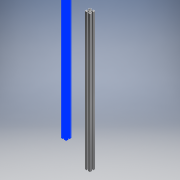
# Autodesk Inventor part: Propile_800
Saved by Autodesk Inventor 2019 (Build 230136000, 136)
## iProperties
Created: 2019-04-15
Part Number: Propile_800
Material: 알루미늄 6061
Document SubType Name: Modeling
Designer: hinmo
Density: 2.7 g/cm^3
Appearance: 알루미늄 - 평지
Mass: 694.099 g
Surface Area: 2965.78 cm^2
Volume: 257.074 cm^3
Author: hinmo
Autodesk Inventor part; units mm, degrees
ref_plane "YZ Plane" through (0, 0, 0) normal (1, 0, 0) x (0, 1, 0)
ref_plane "XZ Plane" through (0, 0, 0) normal (0, 1, 0) x (-1, 0, 0)
ref_plane "XY Plane" through (0, 0, 0) normal (0, 0, 1) x (1, 0, 0)
sketch "스케치1" plane through (0, 0, 0) normal (0, 1, 0) x (-1, 0, 0)
  line L0 (15, 15) -> (-15, -15) construction
  line L1 (-15, 15) -> (15, -15) construction
  line L2 (10, 10) -> (-10, -10) construction
  line L3 (-10, 10) -> (10, -10) construction
  circle A0 centre (-10, -10) radius 3
  arc A1 (-15, -13.5) -> (-13.5, -15) centre (-13.5, -13.5) ccw
  arc A2 (-13.5, 15) -> (-15, 13.5) centre (-13.5, 13.5) ccw
  arc A3 (15, 13.5) -> (13.5, 15) centre (13.5, 13.5) ccw
  arc A4 (13.5, -15) -> (15, -13.5) centre (13.5, -13.5) ccw
  line L4 (-7, -7) -> (-13, -13) construction
  line L5 (-13, -7) -> (-7, -13) construction
  line L6 (-7.5303, -6.4697) -> (-13.5303, -12.4697)
  line L7 (-13.5303, -12.4697) -> (-12.4697, -13.5303)
  line L8 (-12.4697, -13.5303) -> (-6.4697, -7.5303)
  line L9 (-6.4697, -7.5303) -> (-7.5303, -6.4697)
  line L10 (-7.5303, -6.4697) -> (-12.4697, -13.5303) construction
  line L11 (-13.5303, -12.4697) -> (-6.4697, -7.5303) construction
  line L12 (-13.5303, -7.5303) -> (-7.5303, -13.5303)
  line L13 (-7.5303, -13.5303) -> (-6.4697, -12.4697)
  line L14 (-6.4697, -12.4697) -> (-12.4697, -6.4697)
  line L15 (-12.4697, -6.4697) -> (-13.5303, -7.5303)
  line L16 (-13.5303, -7.5303) -> (-6.4697, -12.4697) construction
  line L17 (-7.5303, -13.5303) -> (-12.4697, -6.4697) construction
  circle A5 centre (-10, 10) radius 3
  line L18 (-7, 13) -> (-13, 7) construction
  line L19 (-13, 13) -> (-7, 7) construction
  line L20 (-7.5303, 13.5303) -> (-13.5303, 7.5303)
  line L21 (-13.5303, 7.5303) -> (-12.4697, 6.4697)
  line L22 (-12.4697, 6.4697) -> (-6.4697, 12.4697)
  line L23 (-6.4697, 12.4697) -> (-7.5303, 13.5303)
  line L24 (-7.5303, 13.5303) -> (-12.4697, 6.4697) construction
  line L25 (-13.5303, 7.5303) -> (-6.4697, 12.4697) construction
  line L26 (-13.5303, 12.4697) -> (-7.5303, 6.4697)
  line L27 (-7.5303, 6.4697) -> (-6.4697, 7.5303)
  line L28 (-6.4697, 7.5303) -> (-12.4697, 13.5303)
  line L29 (-12.4697, 13.5303) -> (-13.5303, 12.4697)
  circle A6 centre (10, 10) radius 3
  line L30 (13, 13) -> (7, 7) construction
  line L31 (7, 13) -> (13, 7) construction
  line L32 (12.4697, 13.5303) -> (6.4697, 7.5303)
  line L33 (6.4697, 7.5303) -> (7.5303, 6.4697)
  line L34 (7.5303, 6.4697) -> (13.5303, 12.4697)
  line L35 (13.5303, 12.4697) -> (12.4697, 13.5303)
  line L36 (12.4697, 13.5303) -> (7.5303, 6.4697) construction
  line L37 (6.4697, 7.5303) -> (13.5303, 12.4697) construction
  line L38 (6.4697, 12.4697) -> (12.4697, 6.4697)
  line L39 (12.4697, 6.4697) -> (13.5303, 7.5303)
  line L40 (13.5303, 7.5303) -> (7.5303, 13.5303)
  line L41 (7.5303, 13.5303) -> (6.4697, 12.4697)
  line L42 (6.4697, 12.4697) -> (13.5303, 7.5303) construction
  line L43 (12.4697, 6.4697) -> (7.5303, 13.5303) construction
  circle A7 centre (10, -10) radius 3
  line L44 (13, -7) -> (7, -13) construction
  line L45 (7, -7) -> (13, -13) construction
  line L46 (12.4697, -6.4697) -> (6.4697, -12.4697)
  line L47 (6.4697, -12.4697) -> (7.5303, -13.5303)
  line L48 (7.5303, -13.5303) -> (13.5303, -7.5303)
  line L49 (13.5303, -7.5303) -> (12.4697, -6.4697)
  line L50 (12.4697, -6.4697) -> (7.5303, -13.5303) construction
  line L51 (6.4697, -12.4697) -> (13.5303, -7.5303) construction
  line L52 (6.4697, -7.5303) -> (12.4697, -13.5303)
  line L53 (12.4697, -13.5303) -> (13.5303, -12.4697)
  line L54 (13.5303, -12.4697) -> (7.5303, -6.4697)
  line L55 (7.5303, -6.4697) -> (6.4697, -7.5303)
  line L56 (6.4697, -7.5303) -> (13.5303, -12.4697) construction
  line L57 (12.4697, -13.5303) -> (7.5303, -6.4697) construction
  line L58 (-3.15, -15) -> (-3.15, -12.5)
  line L59 (-3.15, -12.5) -> (-5.1, -12.5)
  line L60 (0, -4.5) -> (-3.435, -4.5)
  arc A8 (-3.435, -4.5) -> (-6.0787, -8.8068) centre (0.5972, -9.94) ccw
  line L61 (-5.1, -12.5) -> (-6.0787, -8.8068)
  line L62 (3.15, -15) -> (3.15, -12.5)
  line L63 (3.15, -12.5) -> (5.1, -12.5)
  line L64 (0, -4.5) -> (3.435, -4.5)
  arc A9 (6.0787, -8.8068) -> (3.435, -4.5) centre (-0.5972, -9.94) ccw
  line L65 (5.1, -12.5) -> (6.0787, -8.8068)
  line L66 (0, -4.5) -> (-0.5, -4.5)
  line L67 (-0.5, -4.5) -> (0.5, -4.5)
  line L68 (0.5, -4.5) -> (0, -4)
  line L69 (-0.5, -4.5) -> (0, -4)
  line L70 (3.15, 15) -> (3.15, 12.5)
  line L71 (3.15, 12.5) -> (5.1, 12.5)
  line L72 (0, 4.5) -> (3.435, 4.5)
  arc A10 (3.435, 4.5) -> (6.0787, 8.8068) centre (-0.5972, 9.94) ccw
  line L73 (5.1, 12.5) -> (6.0787, 8.8068)
  line L74 (0, 4.5) -> (-3.435, 4.5)
  arc A11 (-6.0787, 8.8068) -> (-3.435, 4.5) centre (0.5972, 9.94) ccw
  line L75 (-5.1, 12.5) -> (-6.0787, 8.8068)
  line L76 (-3.15, 12.5) -> (-5.1, 12.5)
  line L77 (-3.15, 15) -> (-3.15, 12.5)
  line L78 (0, 4.5) -> (0.5, 4.5)
  line L79 (0.5, 4.5) -> (-0.5, 4.5)
  line L80 (-0.5, 4.5) -> (0, 4)
  line L81 (0.5, 4.5) -> (0, 4)
  line L82 (-15, 3.15) -> (-12.5, 3.15)
  line L83 (-12.5, 3.15) -> (-12.5, 5.1)
  line L84 (-4.5, 0) -> (-4.5, 3.435)
  arc A12 (-4.5, 3.435) -> (-8.8068, 6.0787) centre (-9.94, -0.5972) ccw
  line L85 (-12.5, 5.1) -> (-8.8068, 6.0787)
  line L86 (-4.5, 0) -> (-4.5, -3.435)
  arc A13 (-8.8068, -6.0787) -> (-4.5, -3.435) centre (-9.94, 0.5972) ccw
  line L87 (-12.5, -5.1) -> (-8.8068, -6.0787)
  line L88 (-12.5, -3.15) -> (-12.5, -5.1)
  line L89 (-15, -3.15) -> (-12.5, -3.15)
  line L90 (-4.5, 0) -> (-4.5, 0.5)
  line L91 (-4.5, 0.5) -> (-4.5, -0.5)
  line L92 (-4.5, -0.5) -> (-4, 0)
  line L93 (-4.5, 0.5) -> (-4, 0)
  line L94 (15, -3.15) -> (12.5, -3.15)
  line L95 (12.5, -3.15) -> (12.5, -5.1)
  line L96 (4.5, 0) -> (4.5, -3.435)
  arc A14 (4.5, -3.435) -> (8.8068, -6.0787) centre (9.94, 0.5972) ccw
  line L97 (12.5, -5.1) -> (8.8068, -6.0787)
  line L98 (4.5, 0) -> (4.5, 3.435)
  arc A15 (8.8068, 6.0787) -> (4.5, 3.435) centre (9.94, -0.5972) ccw
  line L99 (12.5, 5.1) -> (8.8068, 6.0787)
  line L100 (12.5, 3.15) -> (12.5, 5.1)
  line L101 (15, 3.15) -> (12.5, 3.15)
  line L102 (4.5, 0) -> (4.5, -0.5)
  line L103 (4.5, -0.5) -> (4.5, 0.5)
  line L104 (-3.0303, -1.9697) -> (-1.9697, -3.0303)
  line L105 (3.0303, 1.9697) -> (1.9697, 3.0303)
  line L106 (1.9697, 3.0303) -> (-1.9697, -3.0303) construction
  line L107 (-3.0303, -1.9697) -> (3.0303, 1.9697) construction
  line L108 (3.0303, -1.9697) -> (1.9697, -3.0303)
  line L109 (-3.0303, 1.9697) -> (-1.9697, 3.0303)
  line L110 (-1.9697, 3.0303) -> (1.9697, -3.0303) construction
  line L111 (3.0303, -1.9697) -> (-3.0303, 1.9697) construction
  line L112 (-1.9697, -3.0303) -> (-1.3624, -2.0961)
  line L113 (-3.0303, -1.9697) -> (-2.0961, -1.3624)
  line L114 (-3.0303, 1.9697) -> (-2.0961, 1.3624)
  line L115 (-1.9697, 3.0303) -> (-1.3624, 2.0961)
  line L116 (1.9697, 3.0303) -> (1.3624, 2.0961)
  line L117 (3.0303, 1.9697) -> (2.0961, 1.3624)
  line L118 (1.9697, -3.0303) -> (1.3624, -2.0961)
  line L119 (3.0303, -1.9697) -> (2.0961, -1.3624)
  arc A16 (-2.0961, 1.3624) -> (-2.0961, -1.3624) centre (0, 0) ccw
  arc A17 (1.3624, 2.0961) -> (-1.3624, 2.0961) centre (0, 0) ccw
  arc A18 (-1.3624, -2.0961) -> (1.3624, -2.0961) centre (0, 0) ccw
  arc A19 (2.0961, -1.3624) -> (2.0961, 1.3624) centre (0, 0) ccw
  line L120 (-7, 10) -> (-10, 10)
  line L121 (-10, 10) -> (-10, 7)
  line L122 (-10, -7) -> (-10, -10)
  line L123 (-10, -10) -> (-7, -10)
  line L124 (7, -10) -> (10, -10)
  line L125 (10, -10) -> (10, -7)
  line L126 (-13.5, -15) -> (-3.15, -15)
  line L127 (3.15, -15) -> (13.5, -15)
  line L128 (-15, 13.5) -> (-15, 3.15)
  line L129 (-15, -3.15) -> (-15, -13.5)
  line L130 (13.5, 15) -> (3.15, 15)
  line L131 (-3.15, 15) -> (-13.5, 15)
  line L132 (15, -13.5) -> (15, -3.15)
  line L133 (15, 3.15) -> (15, 13.5)
  line L134 (4.5, 0) -> (4.5, -0.5)
  line L135 (4.5, -0.5) -> (4, 0)
  line L136 (4, 0) -> (4.5, 0.5)
  point P0 (0, 0)
  point P1 (-13.5, 6.5)
  point P2 (6.5, 6.5)
  point P3 (6.5, -13.5)
  dimension "d0" = 30
  dimension "d1" = 30
  dimension "d3" = 20
  dimension "d4" = 20
  dimension "d5" = 6
  dimension "d9" = 1.5
  dimension "d10" = 6
  dimension "d11" = 1.5
  dimension "d12" = 1.5
  dimension "d13" = 6
  dimension "d14" = 6
  dimension "d15" = 1.5
  dimension "d16" = 1.5
  dimension "d17" = 6
  dimension "d18" = 6
  dimension "d19" = 1.5
  dimension "d20" = 1.5
  dimension "d21" = 6
  dimension "d22" = 6
  dimension "d23" = 1.5
  dimension "d24" = 1.5
  dimension "d26" = 2.5
  dimension "d27" = 1.95
  dimension "d31" = 3.435
  dimension "d34" = 0.5
  dimension "d35" = 1
  dimension "d37" = 2.5
  dimension "d38" = 1.95
  dimension "d40" = 3.435
  dimension "d41" = 0.5
  dimension "d42" = 1
  dimension "d44" = 2.5
  dimension "d45" = 1.95
  dimension "d47" = 3.435
  dimension "d48" = 0.5
  dimension "d49" = 1
  dimension "d51" = 2.5
  dimension "d52" = 1.95
  dimension "d54" = 3.435
  dimension "d55" = 0.5
  dimension "d56" = 1
  dimension "d57" = 0.5
  constraints: 274 end point, 38 parallel, 38 point on circle, 31 midpoint, 24 perpendicular, 20 centre point, 17 point on line, 16 tangent, 5 coincident, 4 horizontal, 3 equal radius, 1 collinear
  measures "d0" distance of L1.end L0.end
  measures "d1" distance of L0.end L1.start
  measures "d3" distance of L3.end L2.end
  measures "d4" distance of L2.end L3.start
  measures "d5" diameter of A0
  measures "d9" radius of A1
  measures "d10" distance of L4.end L5.start
  measures "d11" distance of L7.end L6.end
  measures "d12" distance of L13.end L12.end
  measures "d13" diameter of A5
  measures "d14" distance of L18.end L19.start
  measures "d15" distance of L22.start L25.start
  measures "d16" distance of L27.end L27.start
  measures "d17" diameter of A6
  measures "d18" distance of L30.end L31.start
  measures "d19" distance of L34.start L37.start
  measures "d20" distance of L39.end L39.start
  measures "d21" diameter of A7
  measures "d22" distance of L44.end L45.start
  measures "d23" distance of L48.start L51.start
  measures "d24" distance of L53.end L53.start
  measures "d26" distance of L58.start L58.end
  measures "d27" distance of L58.end L59.end
  measures "d31" distance of L60.start L60.end
  measures "d34" distance of L60.start L66.end
  measures "d35" distance of L66.end L67.end
  measures "d37" distance of L70.start L71.start
  measures "d38" distance of L71.start L73.start
  measures "d40" distance of L72.start L72.end
  measures "d41" distance of L72.start L79.start
  measures "d42" distance of L79.start L79.end
  measures "d44" distance of L82.start L83.start
  measures "d45" distance of L83.start L85.start
  measures "d47" distance of L90.start L84.end
  measures "d48" distance of L90.start L90.end
  measures "d49" distance of L90.end L91.end
  measures "d51" distance of L94.start L95.start
  measures "d52" distance of L95.start L95.end
  measures "d54" distance of L98.start L96.end
  measures "d55" distance of L98.start L103.start
  measures "d56" distance of L103.start L103.end
  measures "d57" distance of L98.start L103.start
extrude "돌출1" add sketch "스케치1" along normal blind 800 contours L129 L89 L88 L87 A13 L86 L92 L93 L84 A12 L85 L83 L82 L128 A2 L131 L77 L76 L75 A11 L74 L80 L81 L72 A10 L73 L71 L70 L130 A3 L133 L101 L100 L99 A15 L98 L136 L135 L96 A14 L97 L95 L94 L132 A4 L127 L62 L63 L65 A9 L64 L68 L69 L60 A8 L61 L59 L58 L126 A1
fillet "모깎기1" radius 1 8 edges at (15, 400, -3.15) (-3.15, 400, -15) (15, 400, 3.15) (3.15, 400, 15) (-3.15, 400, 15) (-15, 400, -3.15) (-15, 400, 3.15) (3.15, 400, -15)
